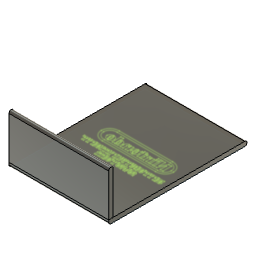
Nintendo Entertainment System Bookend (Autodesk Fusion 360 design; units mm, degrees)
Autodesk Fusion 360 part; units mm, degrees
sketch "Sketch1" plane through (0, 0, 0) normal (0, 0, 1) x (1, 0, 0)
  line L0 (0, 0) -> (67, 0)
  line L1 (67, 0) -> (67, 90)
  line L2 (67, 90) -> (0, 90)
  line L3 (0, 90) -> (0, 0)
  line L4 (0, 0) -> (67, 0)
  line L5 (67, 0) -> (67, -3)
  line L6 (67, -3) -> (0, -3)
  line L7 (0, -3) -> (0, 0)
  dimension "d1" = 67
  dimension "d2" = 90
  dimension "d3" = 67
  dimension "d4" = 3
  constraint horizontal L0
  constraint vertical L1
  constraint horizontal L2
  constraint vertical L3
  constraint coincident L0.start L3.end
  constraint horizontal L4
  constraint vertical L5
  constraint horizontal L6
  constraint vertical L7
  measures "d1" distance of L0.start L0.end
  measures "d2" distance of L0.start L2.end
  measures "d3" distance of L0.start L0.end
  measures "d4" distance of L0.start L6.end
extrude "Extrude1" add sketch "Sketch1" against normal blind 3 makes body 1
extrude "Extrude2" add sketch "Sketch1" along normal blind 30 separate body contours L0 L4 L5 L6 L7 makes body 2
fillet "Fillet1" radius 1.5 1 edges at (33.5, -3, -3) on bodies 1
fillet "Fillet2" radius 1.5 3 edges at (33.5, 90, -3) (33.5, -3, 30) (33.5, 0, 30) on bodies 1 2
fillet "Fillet3" radius 1.5 1 edges at (33.5, 90, 0) on bodies 1
sketch "Sketch2" plane through (0, 0, -3) normal (0, 0, -1) x (1, 0, 0)
  line L0 (0, -88.5) -> (67, -88.5)
  line L1 (67, -88.5) -> (67, 1.5)
  line L2 (67, 1.5) -> (0, 1.5)
  line L3 (0, 1.5) -> (0, -88.5)
  line L4 (53.2046, -41.1196) -> (56.3109, -41.1196)
  line L5 (56.3109, -41.1196) -> (56.3109, -38.078)
  line L6 (56.3109, -38.078) -> (55.3464, -38.078)
  line L7 (55.3464, -38.078) -> (55.3464, -40.1128)
  spline S0 degree 3 poles (55.3464, -40.1128) (55.3464, -40.2417) (55.2397, -40.3486) (55.111, -40.3486) knots 0 0 0 0 1 1 1 1
  line L8 (55.111, -40.3486) -> (53.4406, -40.3486)
  spline S1 degree 3 poles (53.4406, -40.3486) (53.3124, -40.3486) (53.2046, -40.2417) (53.2046, -40.1128) knots 0 0 0 0 1 1 1 1
  line L9 (53.2046, -40.1128) -> (53.2046, -38.078)
  line L10 (53.2046, -38.078) -> (52.2413, -38.078)
  line L11 (52.2413, -38.078) -> (52.2413, -40.1128)
  spline S2 degree 2 poles (52.2413, -40.1128) (52.1124, -41.1196) (53.2046, -41.1196) knots 0 0 0 1 1 1
  line L12 (26.3683, -41.1196) -> (29.4748, -41.1196)
  line L13 (29.4748, -41.1196) -> (29.4748, -38.078)
  line L14 (29.4748, -38.078) -> (28.4897, -38.078)
  line L15 (28.4897, -38.078) -> (28.4897, -40.1128)
  spline S3 degree 3 poles (28.4897, -40.1128) (28.4897, -40.2417) (28.3819, -40.3486) (28.2749, -40.3486) knots 0 0 0 0 1 1 1 1
  line L16 (28.2749, -40.3486) -> (26.6038, -40.3486)
  spline S4 degree 3 poles (26.6038, -40.3486) (26.4759, -40.3486) (26.3683, -40.2417) (26.3683, -40.1128) knots 0 0 0 0 1 1 1 1
  line L17 (26.3683, -40.1128) -> (26.3683, -38.078)
  line L18 (26.3683, -38.078) -> (25.4052, -38.078)
  line L19 (25.4052, -38.078) -> (25.4052, -40.1128)
  spline S5 degree 2 poles (25.4052, -40.1128) (25.2768, -41.1196) (26.3683, -41.1196) knots 0 0 0 1 1 1
  line L20 (11.74, -41.1196) -> (14.846, -41.1196)
  line L21 (14.846, -41.1196) -> (14.846, -38.078)
  line L22 (14.846, -38.078) -> (13.8814, -38.078)
  line L23 (13.8814, -38.078) -> (13.8814, -40.1128)
  spline S6 degree 3 poles (13.8814, -40.1128) (13.8814, -40.2417) (13.7753, -40.3486) (13.6459, -40.3486) knots 0 0 0 0 1 1 1 1
  line L24 (13.6459, -40.3486) -> (11.9756, -40.3486)
  spline S7 degree 3 poles (11.9756, -40.3486) (11.8477, -40.3486) (11.74, -40.2417) (11.74, -40.1128) knots 0 0 0 0 1 1 1 1
  line L25 (11.74, -40.1128) -> (11.74, -38.078)
  line L26 (11.74, -38.078) -> (10.7763, -38.078)
  line L27 (10.7763, -38.078) -> (10.7763, -40.1128)
  spline S8 degree 2 poles (10.7763, -40.1128) (10.6485, -41.1196) (11.74, -41.1196) knots 0 0 0 1 1 1
  line L28 (51.8126, -40.3486) -> (50.7419, -40.3486)
  spline S9 degree 3 poles (50.7419, -40.3486) (50.6348, -40.3486) (50.5059, -40.2417) (50.5059, -40.1128) knots 0 0 0 0 1 1 1 1
  line L29 (50.5059, -40.1128) -> (50.5059, -38.078)
  line L30 (50.5059, -38.078) -> (49.4786, -38.078)
  line L31 (49.4786, -38.078) -> (49.4786, -40.1128)
  spline S10 degree 3 poles (49.4786, -40.1128) (49.4786, -40.2417) (49.3709, -40.3486) (49.2427, -40.3486) knots 0 0 0 0 1 1 1 1
  line L32 (49.2427, -40.3486) -> (48.172, -40.3486)
  line L33 (48.172, -40.3486) -> (48.172, -41.1196)
  line L34 (48.172, -41.1196) -> (51.8126, -41.1196)
  line L35 (51.8126, -41.1196) -> (51.8126, -40.3486)
  line L36 (10.3698, -41.1196) -> (10.3698, -40.3486)
  line L37 (10.3698, -40.3486) -> (9.2984, -40.3486)
  spline S11 degree 3 poles (9.2984, -40.3486) (9.1706, -40.3486) (9.0628, -40.2417) (9.0628, -40.1128) knots 0 0 0 0 1 1 1 1
  line L38 (9.0628, -40.1128) -> (9.0628, -38.078)
  line L39 (9.0628, -38.078) -> (7.9914, -38.078)
  line L40 (7.9914, -38.078) -> (7.9914, -40.1128)
  spline S12 degree 3 poles (7.9914, -40.1128) (7.9914, -40.2417) (7.9067, -40.3486) (7.7782, -40.3486) knots 0 0 0 0 1 1 1 1
  line L41 (7.7782, -40.3486) -> (6.7068, -40.3486)
  line L42 (6.7068, -40.3486) -> (6.7068, -41.1196)
  line L43 (6.7068, -41.1196) -> (10.3698, -41.1196)
  line L44 (39.5829, -40.3486) -> (38.5121, -40.3486)
  spline S13 degree 3 poles (38.5121, -40.3486) (38.3839, -40.3486) (38.2763, -40.2417) (38.2763, -40.1128) knots 0 0 0 0 1 1 1 1
  line L45 (38.2763, -40.1128) -> (38.2763, -38.078)
  line L46 (38.2763, -38.078) -> (37.2063, -38.078)
  line L47 (37.2063, -38.078) -> (37.2063, -40.1128)
  spline S14 degree 3 poles (37.2063, -40.1128) (37.2063, -40.2417) (37.0985, -40.3486) (36.9696, -40.3486) knots 0 0 0 0 1 1 1 1
  line L48 (36.9696, -40.3486) -> (35.8996, -40.3486)
  line L49 (35.8996, -40.3486) -> (35.8996, -41.1196)
  line L50 (35.8996, -41.1196) -> (39.5829, -41.1196)
  line L51 (39.5829, -41.1196) -> (39.5829, -40.3486)
  line L52 (31.1446, -41.1196) -> (30.1168, -41.1196)
  line L53 (30.1168, -41.1196) -> (30.1168, -38.0781)
  line L54 (30.1168, -38.0781) -> (31.1446, -38.0781)
  line L55 (31.1446, -38.0781) -> (31.1446, -41.1196)
  line L56 (32.7941, -39.6198) -> (34.528, -39.6198)
  line L57 (34.528, -39.6198) -> (34.528, -40.1555)
  spline S15 degree 3 poles (34.528, -40.1555) (34.528, -40.2417) (34.3998, -40.3486) (34.3359, -40.3486) knots 0 0 0 0 1 1 1 1
  line L58 (34.3359, -40.3486) -> (33.0296, -40.3486)
  spline S16 degree 3 poles (33.0296, -40.3486) (32.8802, -40.3486) (32.7941, -40.2417) (32.7941, -40.1555) knots 0 0 0 0 1 1 1 1
  line L59 (32.7941, -40.1555) -> (32.7941, -39.6198)
  line L60 (32.8156, -41.1196) -> (34.5075, -41.1196)
  spline S17 degree 2 poles (34.5075, -41.1196) (35.5998, -41.1196) (35.5136, -40.1128) knots 0 0 0 1 1 1
  line L61 (35.5136, -40.1128) -> (35.5136, -38.078)
  line L62 (35.5136, -38.078) -> (34.528, -38.078)
  line L63 (34.528, -38.078) -> (34.528, -38.8485)
  line L64 (34.528, -38.8485) -> (32.7941, -38.8485)
  line L65 (32.7941, -38.8485) -> (32.7941, -38.078)
  line L66 (32.7941, -38.078) -> (31.8095, -38.078)
  line L67 (31.8095, -38.078) -> (31.8095, -40.1128)
  spline S18 degree 2 poles (31.8095, -40.1128) (31.681, -41.1196) (32.8156, -41.1196) knots 0 0 0 1 1 1
  spline S19 degree 3 poles (40.9539, -39.8553) (40.9539, -39.706) (41.0177, -39.6198) (41.1466, -39.6198) knots 0 0 0 0 1 1 1 1
  line L68 (41.1466, -39.6198) -> (42.5603, -39.6198)
  spline S20 degree 3 poles (42.5603, -39.6198) (42.6242, -39.6198) (42.7096, -39.706) (42.7096, -39.8553) knots 0 0 0 0 1 1 1 1
  line L69 (42.7096, -39.8553) -> (42.7096, -40.1555)
  spline S21 degree 3 poles (42.7096, -40.1555) (42.7096, -40.2844) (42.6242, -40.3913) (42.496, -40.3913) knots 0 0 0 0 1 1 1 1
  line L70 (42.496, -40.3913) -> (41.1466, -40.3913)
  spline S22 degree 3 poles (41.1466, -40.3913) (41.0177, -40.3913) (40.9539, -40.3278) (40.9539, -40.1555) knots 0 0 0 0 1 1 1 1
  line L71 (40.9539, -40.1555) -> (40.9539, -39.8553)
  line L72 (40.975, -41.1196) -> (43.7165, -41.1196)
  line L73 (43.7165, -41.1196) -> (43.7165, -38.078)
  line L74 (43.7165, -38.078) -> (42.7096, -38.078)
  line L75 (42.7096, -38.078) -> (42.7096, -38.6568)
  spline S23 degree 3 poles (42.7096, -38.6568) (42.7096, -38.7852) (42.6242, -38.8485) (42.496, -38.8485) knots 0 0 0 0 1 1 1 1
  line L76 (42.496, -38.8485) -> (41.1466, -38.8485)
  spline S24 degree 3 poles (41.1466, -38.8485) (41.0826, -38.8485) (40.9539, -38.7415) (40.9539, -38.6568) knots 0 0 0 0 1 1 1 1
  line L77 (40.9539, -38.6568) -> (40.9539, -38.078)
  line L78 (40.9539, -38.078) -> (39.9904, -38.078)
  line L79 (39.9904, -38.078) -> (39.9904, -38.5485)
  spline S25 degree 2 poles (39.9904, -38.5485) (39.9043, -38.9784) (40.3542, -39.2779) knots 0 0 0 1 1 1
  spline S26 degree 3 poles (40.3542, -39.2779) (40.0543, -39.4919) (39.947, -39.8123) (39.9255, -40.0061) knots 0 0 0 0 1 1 1 1
  spline S27 degree 2 poles (39.9255, -40.0061) (39.9043, -40.0916) (39.9043, -40.1555) knots 0 0 0 1 1 1
  spline S28 degree 2 poles (39.9043, -40.1555) (39.9043, -41.1196) (40.975, -41.1196) knots 0 0 0 1 1 1
  spline S29 degree 2 poles (60.3589, -39.0848) (60.4657, -38.078) (59.3518, -38.078) knots 0 0 0 1 1 1
  line L80 (59.3518, -38.078) -> (56.9529, -38.078)
  line L81 (56.9529, -38.078) -> (56.9529, -38.8485)
  line L82 (56.9529, -38.8485) -> (59.1808, -38.8485)
  spline S30 degree 3 poles (59.1808, -38.8485) (59.3306, -38.8485) (59.4595, -38.9784) (59.4595, -39.1057) knots 0 0 0 0 1 1 1 1
  spline S31 degree 3 poles (59.4595, -39.1057) (59.4595, -39.2556) (59.3518, -39.3418) (59.1808, -39.3418) knots 0 0 0 0 1 1 1 1
  line L83 (59.1808, -39.3418) -> (57.0811, -39.3418)
  line L84 (57.0811, -39.3418) -> (57.0811, -39.8769)
  line L85 (57.0811, -39.8769) -> (59.2236, -39.8769)
  spline S32 degree 3 poles (59.2236, -39.8769) (59.3518, -39.8769) (59.4595, -39.9839) (59.4595, -40.1128) knots 0 0 0 0 1 1 1 1
  spline S33 degree 3 poles (59.4595, -40.1128) (59.4595, -40.2417) (59.3518, -40.3486) (59.2236, -40.3486) knots 0 0 0 0 1 1 1 1
  line L86 (59.2236, -40.3486) -> (56.9529, -40.3486)
  line L87 (56.9529, -40.3486) -> (56.9529, -41.1196)
  line L88 (56.9529, -41.1196) -> (60.3589, -41.1196)
  line L89 (60.3589, -41.1196) -> (60.3589, -39.0848)
  spline S34 degree 2 poles (47.7217, -39.0848) (47.8722, -38.078) (46.7577, -38.078) knots 0 0 0 1 1 1
  line L90 (46.7577, -38.078) -> (44.3588, -38.078)
  line L91 (44.3588, -38.078) -> (44.3588, -38.8485)
  line L92 (44.3588, -38.8485) -> (46.5867, -38.8485)
  spline S35 degree 3 poles (46.5867, -38.8485) (46.7372, -38.8485) (46.8654, -38.9784) (46.8654, -39.1057) knots 0 0 0 0 1 1 1 1
  spline S36 degree 3 poles (46.8654, -39.1057) (46.8654, -39.2556) (46.7372, -39.3418) (46.5867, -39.3418) knots 0 0 0 0 1 1 1 1
  line L93 (46.5867, -39.3418) -> (44.4877, -39.3418)
  line L94 (44.4877, -39.3418) -> (44.4877, -39.8769)
  line L95 (44.4877, -39.8769) -> (46.5867, -39.8769)
  spline S37 degree 3 poles (46.5867, -39.8769) (46.7372, -39.8769) (46.8654, -39.9839) (46.8654, -40.1128) knots 0 0 0 0 1 1 1 1
  spline S38 degree 3 poles (46.8654, -40.1128) (46.8654, -40.2417) (46.7372, -40.3486) (46.5867, -40.3486) knots 0 0 0 0 1 1 1 1
  line L96 (46.5867, -40.3486) -> (44.3588, -40.3486)
  line L97 (44.3588, -40.3486) -> (44.3588, -41.1196)
  line L98 (44.3588, -41.1196) -> (47.7217, -41.1196)
  line L99 (47.7217, -41.1196) -> (47.7217, -39.0848)
  spline S39 degree 2 poles (18.8509, -39.0848) (18.9586, -38.078) (17.8656, -38.078) knots 0 0 0 1 1 1
  line L100 (17.8656, -38.078) -> (15.4456, -38.078)
  line L101 (15.4456, -38.078) -> (15.4456, -38.8485)
  line L102 (15.4456, -38.8485) -> (17.6948, -38.8485)
  spline S40 degree 3 poles (17.6948, -38.8485) (17.8232, -38.8485) (17.9517, -38.9784) (17.9517, -39.1057) knots 0 0 0 0 1 1 1 1
  spline S41 degree 3 poles (17.9517, -39.1057) (17.9517, -39.2556) (17.8656, -39.3418) (17.7156, -39.3418) knots 0 0 0 0 1 1 1 1
  line L103 (17.7156, -39.3418) -> (15.6172, -39.3418)
  line L104 (15.6172, -39.3418) -> (15.6172, -39.8769)
  line L105 (15.6172, -39.8769) -> (17.7156, -39.8769)
  spline S42 degree 3 poles (17.7156, -39.8769) (17.8656, -39.8769) (17.9517, -39.9839) (17.9517, -40.1128) knots 0 0 0 0 1 1 1 1
  spline S43 degree 3 poles (17.9517, -40.1128) (17.9517, -40.2417) (17.8656, -40.3486) (17.7156, -40.3486) knots 0 0 0 0 1 1 1 1
  line L106 (17.7156, -40.3486) -> (15.4456, -40.3486)
  line L107 (15.4456, -40.3486) -> (15.4456, -41.1196)
  line L108 (15.4456, -41.1196) -> (18.8509, -41.1196)
  line L109 (18.8509, -41.1196) -> (18.8509, -39.0848)
  line L110 (20.45, -41.1156) -> (24.7558, -41.1156)
  line L111 (24.7558, -41.1156) -> (24.7558, -38.0745)
  line L112 (24.7558, -38.0745) -> (23.856, -38.0745)
  line L113 (23.856, -38.0745) -> (23.856, -40.1088)
  spline S44 degree 3 poles (23.856, -40.1088) (23.856, -40.2369) (23.749, -40.3443) (23.6204, -40.3443) knots 0 0 0 0 1 1 1 1
  line L114 (23.6204, -40.3443) -> (22.8928, -40.3443)
  spline S45 degree 3 poles (22.8928, -40.3443) (22.7638, -40.3443) (22.6561, -40.2369) (22.6561, -40.1088) knots 0 0 0 0 1 1 1 1
  line L115 (22.6561, -40.1088) -> (22.6561, -38.0745)
  line L116 (22.6561, -38.0745) -> (21.6499, -38.0745)
  line L117 (21.6499, -38.0745) -> (21.6499, -40.1088)
  spline S46 degree 3 poles (21.6499, -40.1088) (21.6499, -40.2369) (21.5638, -40.3443) (21.4143, -40.3443) knots 0 0 0 0 1 1 1 1
  line L118 (21.4143, -40.3443) -> (20.643, -40.3443)
  spline S47 degree 3 poles (20.643, -40.3443) (20.5577, -40.3443) (20.45, -40.2369) (20.45, -40.1088) knots 0 0 0 0 1 1 1 1
  line L119 (20.45, -40.1088) -> (20.4082, -38.0745)
  line L120 (20.4082, -38.0745) -> (19.4445, -38.0745)
  line L121 (19.4445, -38.0745) -> (19.4445, -40.1088)
  spline S48 degree 2 poles (19.4445, -40.1088) (19.316, -41.1156) (20.45, -41.1156) knots 0 0 0 1 1 1
  line L122 (34.143, -36.1081) -> (33.0511, -36.1081)
  spline S49 degree 3 poles (33.0511, -36.1081) (32.9664, -36.1081) (32.8587, -36.0004) (32.8587, -35.8726) knots 0 0 0 0 1 1 1 1
  line L123 (32.8587, -35.8726) -> (32.8587, -33.8382)
  line L124 (32.8587, -33.8382) -> (31.7872, -33.8382)
  line L125 (31.7872, -33.8382) -> (31.7448, -35.8726)
  spline S50 degree 3 poles (31.7448, -35.8726) (31.7448, -36.0004) (31.681, -36.1081) (31.5517, -36.1081) knots 0 0 0 0 1 1 1 1
  line L126 (31.5517, -36.1081) -> (30.4803, -36.1081)
  line L127 (30.4803, -36.1081) -> (30.4803, -36.8787)
  line L128 (30.4803, -36.8787) -> (34.143, -36.8787)
  line L129 (34.143, -36.8787) -> (34.143, -36.1081)
  line L130 (21.7636, -36.8787) -> (26.0681, -36.8787)
  line L131 (26.0681, -36.8787) -> (26.0681, -33.8382)
  line L132 (26.0681, -33.8382) -> (25.169, -33.8382)
  line L133 (25.169, -33.8382) -> (25.169, -35.8726)
  spline S51 degree 3 poles (25.169, -35.8726) (25.169, -36.0004) (25.062, -36.1081) (24.9334, -36.1081) knots 0 0 0 0 1 1 1 1
  line L134 (24.9334, -36.1081) -> (24.2053, -36.1081)
  spline S52 degree 3 poles (24.2053, -36.1081) (24.0774, -36.1081) (23.9704, -36.0004) (23.9704, -35.8726) knots 0 0 0 0 1 1 1 1
  line L135 (23.9704, -35.8726) -> (23.9704, -33.8382)
  line L136 (23.9704, -33.8382) -> (22.9637, -33.8382)
  line L137 (22.9637, -33.8382) -> (22.9637, -35.8726)
  spline S53 degree 3 poles (22.9637, -35.8726) (22.9637, -36.0004) (22.8781, -36.1081) (22.7274, -36.1081) knots 0 0 0 0 1 1 1 1
  line L138 (22.7274, -36.1081) -> (21.9568, -36.1081)
  spline S54 degree 3 poles (21.9568, -36.1081) (21.8707, -36.1081) (21.7636, -36.0004) (21.7636, -35.8726) knots 0 0 0 0 1 1 1 1
  line L139 (21.7636, -35.8726) -> (21.7206, -33.8382)
  line L140 (21.7206, -33.8382) -> (20.7568, -33.8382)
  line L141 (20.7568, -33.8382) -> (20.7568, -35.8726)
  spline S55 degree 2 poles (20.7568, -35.8726) (20.629, -36.8787) (21.7636, -36.8787) knots 0 0 0 1 1 1
  line L142 (38.5549, -36.8787) -> (39.4762, -36.8787)
  line L143 (39.4762, -36.8787) -> (39.4762, -35.7434)
  spline S56 degree 3 poles (39.4762, -35.7434) (39.4762, -35.6161) (39.6044, -35.5085) (39.7111, -35.5085) knots 0 0 0 0 1 1 1 1
  line L144 (39.7111, -35.5085) -> (41.0826, -35.5085)
  spline S57 degree 3 poles (41.0826, -35.5085) (41.2108, -35.5085) (41.3182, -35.6161) (41.3182, -35.7434) knots 0 0 0 0 1 1 1 1
  line L145 (41.3182, -35.7434) -> (41.3182, -36.8787)
  line L146 (41.3182, -36.8787) -> (42.2816, -36.8787)
  line L147 (42.2816, -36.8787) -> (42.2816, -35.7649)
  spline S58 degree 2 poles (42.2816, -35.7649) (42.3886, -34.7379) (41.2748, -34.7379) knots 0 0 0 1 1 1
  line L148 (41.2748, -34.7379) -> (40.9539, -34.7379)
  line L149 (40.9539, -34.7379) -> (40.9539, -33.8382)
  line L150 (40.9539, -33.8382) -> (39.8827, -33.8382)
  line L151 (39.8827, -33.8382) -> (39.8827, -34.7379)
  line L152 (39.8827, -34.7379) -> (39.5189, -34.7379)
  spline S59 degree 2 poles (39.5189, -34.7379) (38.4051, -34.7379) (38.5549, -35.7434) knots 0 0 0 1 1 1
  line L153 (38.5549, -35.7434) -> (38.5549, -36.8787)
  spline S60 degree 2 poles (30.0739, -34.8443) (30.2238, -33.8382) (29.1101, -33.8382) knots 0 0 0 1 1 1
  line L154 (29.1101, -33.8382) -> (26.7115, -33.8382)
  line L155 (26.7115, -33.8382) -> (26.7115, -34.6093)
  line L156 (26.7115, -34.6093) -> (28.9385, -34.6093)
  spline S61 degree 3 poles (28.9385, -34.6093) (29.0886, -34.6093) (29.2177, -34.7164) (29.2177, -34.8665) knots 0 0 0 0 1 1 1 1
  spline S62 degree 3 poles (29.2177, -34.8665) (29.2177, -35.0158) (29.0886, -35.0797) (28.9385, -35.0797) knots 0 0 0 0 1 1 1 1
  line L157 (28.9385, -35.0797) -> (26.8401, -35.0797)
  line L158 (26.8401, -35.0797) -> (26.8401, -35.6161)
  line L159 (26.8401, -35.6161) -> (28.9385, -35.6161)
  spline S63 degree 3 poles (28.9385, -35.6161) (29.0886, -35.6161) (29.2177, -35.7434) (29.2177, -35.8726) knots 0 0 0 0 1 1 1 1
  spline S64 degree 3 poles (29.2177, -35.8726) (29.2177, -36.0004) (29.0886, -36.1081) (28.9385, -36.1081) knots 0 0 0 0 1 1 1 1
  line L160 (28.9385, -36.1081) -> (26.7115, -36.1081)
  line L161 (26.7115, -36.1081) -> (26.7115, -36.8787)
  line L162 (26.7115, -36.8787) -> (30.0739, -36.8787)
  line L163 (30.0739, -36.8787) -> (30.0739, -34.8443)
  line L164 (35.4709, -35.6377) -> (36.9064, -35.6377)
  spline S65 degree 3 poles (36.9064, -35.6377) (37.0773, -35.6377) (37.184, -35.701) (37.184, -35.8504) knots 0 0 0 0 1 1 1 1
  spline S66 degree 3 poles (37.184, -35.8504) (37.184, -35.9802) (37.0773, -36.1081) (36.9491, -36.1081) knots 0 0 0 0 1 1 1 1
  line L165 (36.9491, -36.1081) -> (34.5075, -36.1081)
  line L166 (34.5075, -36.1081) -> (34.5075, -36.8787)
  line L167 (34.5075, -36.8787) -> (37.184, -36.8787)
  spline S67 degree 3 poles (37.184, -36.8787) (37.677, -36.8787) (38.1047, -36.4722) (38.1047, -36.0004) knots 0 0 0 0 1 1 1 1
  spline S68 degree 3 poles (38.1047, -36.0004) (38.1047, -35.3368) (37.677, -35.0797) (37.0985, -35.0797) knots 0 0 0 0 1 1 1 1
  line L168 (37.0985, -35.0797) -> (35.6637, -35.0797)
  spline S69 degree 3 poles (35.6637, -35.0797) (35.5136, -35.0797) (35.3636, -35.0158) (35.3636, -34.8665) knots 0 0 0 0 1 1 1 1
  spline S70 degree 3 poles (35.3636, -34.8665) (35.3636, -34.7379) (35.4709, -34.6093) (35.5998, -34.6093) knots 0 0 0 0 1 1 1 1
  line L169 (35.5998, -34.6093) -> (38.1047, -34.6093)
  line L170 (38.1047, -34.6093) -> (38.1047, -33.8382)
  line L171 (38.1047, -33.8382) -> (35.3636, -33.8382)
  spline S71 degree 3 poles (35.3636, -33.8382) (34.914, -33.8382) (34.4426, -34.2022) (34.4426, -34.7164) knots 0 0 0 0 1 1 1 1
  spline S72 degree 3 poles (34.4426, -34.7164) (34.4426, -35.3368) (34.9356, -35.6377) (35.4709, -35.6377) knots 0 0 0 0 1 1 1 1
  line L172 (43.631, -35.6377) -> (45.023, -35.6377)
  spline S73 degree 3 poles (45.023, -35.6377) (45.1947, -35.6377) (45.3229, -35.701) (45.3229, -35.8504) knots 0 0 0 0 1 1 1 1
  spline S74 degree 3 poles (45.3229, -35.8504) (45.3229, -35.9802) (45.1947, -36.1081) (45.0658, -36.1081) knots 0 0 0 0 1 1 1 1
  line L173 (45.0658, -36.1081) -> (42.6242, -36.1081)
  line L174 (42.6242, -36.1081) -> (42.6242, -36.8787)
  line L175 (42.6242, -36.8787) -> (45.3017, -36.8787)
  spline S75 degree 3 poles (45.3017, -36.8787) (45.8371, -36.8787) (46.2657, -36.4722) (46.2657, -36.0004) knots 0 0 0 0 1 1 1 1
  spline S76 degree 3 poles (46.2657, -36.0004) (46.2657, -35.3368) (45.7943, -35.0797) (45.2162, -35.0797) knots 0 0 0 0 1 1 1 1
  line L176 (45.2162, -35.0797) -> (43.8241, -35.0797)
  spline S77 degree 3 poles (43.8241, -35.0797) (43.6525, -35.0797) (43.5243, -35.0158) (43.5243, -34.8665) knots 0 0 0 0 1 1 1 1
  spline S78 degree 3 poles (43.5243, -34.8665) (43.5243, -34.7379) (43.6525, -34.6093) (43.7813, -34.6093) knots 0 0 0 0 1 1 1 1
  line L177 (43.7813, -34.6093) -> (46.2657, -34.6093)
  line L178 (46.2657, -34.6093) -> (46.2657, -33.8382)
  line L179 (46.2657, -33.8382) -> (43.5243, -33.8382)
  spline S79 degree 3 poles (43.5243, -33.8382) (43.0316, -33.8382) (42.5814, -34.2022) (42.5814, -34.7164) knots 0 0 0 0 1 1 1 1
  spline S80 degree 3 poles (42.5814, -34.7164) (42.5814, -35.3368) (43.0529, -35.6377) (43.631, -35.6377) knots 0 0 0 0 1 1 1 1
  spline S81 degree 3 poles (51.5861, -43.9141) (55.3819, -43.9152) (57.9183, -46.4889) (57.9183, -49.6094) knots 0 0 0 0 1 1 1 1
  spline S82 degree 3 poles (57.9183, -49.6094) (57.9183, -52.7298) (55.3761, -55.3329) (51.5919, -55.3249) knots 0 0 0 0 1 1 1 1
  line L180 (51.5919, -55.3249) -> (15.8311, -55.3249)
  spline S83 degree 3 poles (15.8311, -55.3249) (12.0469, -55.3329) (9.5047, -52.7298) (9.5047, -49.6094) knots 0 0 0 0 1 1 1 1
  spline S84 degree 3 poles (9.5047, -49.6094) (9.5047, -46.4889) (12.0411, -43.9153) (15.8369, -43.9141) knots 0 0 0 0 1 1 1 1
  line L181 (15.8369, -43.9141) -> (51.5861, -43.9141)
  spline S85 degree 3 poles (51.5745, -53.9213) (54.5795, -53.9158) (56.4241, -51.9941) (56.4241, -49.6168) knots 0 0 0 0 1 1 1 1
  spline S86 degree 3 poles (56.4241, -49.6168) (56.4241, -47.24) (54.5911, -45.3024) (51.5745, -45.3129) knots 0 0 0 0 1 1 1 1
  line L182 (51.5745, -45.3129) -> (15.8485, -45.3129)
  spline S87 degree 3 poles (15.8485, -45.3129) (12.8319, -45.303) (10.9982, -47.24) (10.9982, -49.6168) knots 0 0 0 0 1 1 1 1
  spline S88 degree 3 poles (10.9982, -49.6168) (10.9982, -51.9935) (12.8428, -53.9151) (15.8478, -53.9207) knots 0 0 0 0 1 1 1 1
  line L183 (15.8478, -53.9207) -> (51.5745, -53.9213)
  line L184 (49.5717, -52.4118) -> (47.8083, -52.4118)
  line L185 (47.8083, -52.4118) -> (47.8083, -46.7083)
  line L186 (47.8083, -46.7083) -> (49.5691, -46.7083)
  line L187 (49.5691, -46.7083) -> (52.0404, -50.6856)
  line L188 (52.0404, -50.6856) -> (52.0404, -46.7083)
  line L189 (52.0404, -46.7083) -> (53.8064, -46.7083)
  line L190 (53.8064, -46.7083) -> (53.8057, -52.4118)
  line L191 (53.8057, -52.4118) -> (52.0287, -52.4118)
  line L192 (52.0287, -52.4118) -> (49.5704, -48.4344)
  line L193 (49.5704, -48.4344) -> (49.5717, -52.4118)
  line L194 (39.1541, -50.4936) -> (39.1541, -51.0566)
  line L195 (39.1541, -51.0566) -> (38.2208, -51.0573)
  line L196 (38.2208, -51.0573) -> (38.2221, -51.8253)
  line L197 (38.2221, -51.8253) -> (36.5058, -51.8253)
  line L198 (36.5058, -51.8253) -> (36.5058, -51.0579)
  line L199 (36.5058, -51.0579) -> (35.5771, -51.0579)
  line L200 (35.5771, -51.0579) -> (35.5771, -50.4936)
  line L201 (35.5771, -50.4936) -> (36.5058, -50.4936)
  line L202 (36.5058, -50.4936) -> (36.5045, -46.7083)
  line L203 (36.5045, -46.7083) -> (38.2221, -46.7083)
  line L204 (38.2221, -46.7083) -> (38.2215, -50.4936)
  line L205 (38.2215, -50.4936) -> (39.1541, -50.4936)
  line L206 (45.1117, -50.5008) -> (45.1117, -46.7083)
  line L207 (45.1117, -46.7083) -> (46.8267, -46.7083)
  line L208 (46.8267, -46.7083) -> (46.8267, -50.5015)
  line L209 (46.8267, -50.5015) -> (45.1117, -50.5008)
  line L210 (45.1117, -52.4131) -> (45.1117, -51.2473)
  line L211 (45.1117, -51.2473) -> (46.8306, -51.2473)
  line L212 (46.8306, -51.2473) -> (46.8306, -52.4131)
  line L213 (46.8306, -52.4131) -> (45.1117, -52.4131)
  spline S89 degree 2 poles (16.0814, -48.6349) (16.0822, -48.0615) (16.0822, -47.8316) knots 0 0 0 1 1 1
  spline S90 degree 3 poles (16.0822, -47.8316) (16.0822, -47.2268) (16.4394, -46.9773) (16.783, -46.9773) knots 0 0 0 0 1 1 1 1
  spline S91 degree 3 poles (16.783, -46.9773) (17.1272, -46.9773) (17.4857, -47.2268) (17.4857, -47.8316) knots 0 0 0 0 1 1 1 1
  spline S92 degree 2 poles (17.4857, -47.8316) (17.4857, -48.0615) (17.485, -48.6493) knots 0 0 0 1 1 1
  spline S93 degree 2 poles (17.485, -48.6493) (17.4837, -49.2103) (17.4837, -49.4402) knots 0 0 0 1 1 1
  spline S94 degree 3 poles (17.4837, -49.4402) (17.4837, -50.0423) (17.1245, -50.2899) (16.7829, -50.2899) knots 0 0 0 0 1 1 1 1
  spline S95 degree 3 poles (16.7829, -50.2899) (16.4407, -50.2899) (16.0822, -50.0423) (16.0822, -49.4402) knots 0 0 0 0 1 1 1 1
  spline S96 degree 3 poles (16.0822, -49.4402) (16.0822, -49.2103) (16.0829, -48.7851) (16.0809, -48.633) knots 0 0 0 0 1 1 1 1
  line L214 (16.0809, -48.633) -> (16.0814, -48.6349)
  spline S97 degree 3 poles (16.7705, -50.7601) (18.155, -50.7601) (19.2771, -49.8066) (19.2771, -48.6303) knots 0 0 0 0 1 1 1 1
  spline S98 degree 3 poles (19.2771, -48.6303) (19.2771, -47.4541) (18.1544, -46.5006) (16.7705, -46.5006) knots 0 0 0 0 1 1 1 1
  spline S99 degree 3 poles (16.7705, -46.5006) (15.3859, -46.5006) (14.2639, -47.4541) (14.2639, -48.6303) knots 0 0 0 0 1 1 1 1
  spline S100 degree 3 poles (14.2639, -48.6303) (14.2639, -49.8066) (15.3859, -50.7601) (16.7705, -50.7601) knots 0 0 0 0 1 1 1 1
  line L215 (21.5283, -52.4118) -> (19.8355, -52.4118)
  line L216 (19.8355, -52.4118) -> (19.8355, -46.7083)
  line L217 (19.8355, -46.7083) -> (21.5309, -46.7083)
  spline S101 degree 2 poles (21.5309, -46.7083) (21.5317, -46.8924) (21.5317, -46.9277) knots 0 0 0 1 1 1
  spline S102 degree 3 poles (21.5317, -46.9277) (22.188, -46.5156) (22.9286, -46.5163) (23.5053, -46.7853) knots 0 0 0 0 1 1 1 1
  spline S103 degree 3 poles (23.5053, -46.7853) (23.6601, -46.8572) (24.6783, -47.3457) (24.6783, -48.6656) knots 0 0 0 0 1 1 1 1
  spline S104 degree 3 poles (24.6783, -48.6656) (24.6783, -49.6668) (23.7339, -50.7601) (22.4976, -50.6517) knots 0 0 0 0 1 1 1 1
  spline S105 degree 3 poles (22.4976, -50.6517) (22.0907, -50.6158) (21.8014, -50.4675) (21.5271, -50.3134) knots 0 0 0 0 1 1 1 1
  spline S106 degree 2 poles (21.5271, -50.3134) (21.5283, -51.1911) (21.5283, -52.4118) knots 0 0 0 1 1 1
  spline S107 degree 2 poles (21.5159, -48.6238) (21.5159, -49.0993) (21.5159, -49.3017) knots 0 0 0 1 1 1
  spline S108 degree 3 poles (21.5159, -49.3017) (21.5159, -49.8882) (21.9208, -50.0378) (22.1873, -50.0378) knots 0 0 0 0 1 1 1 1
  spline S109 degree 3 poles (22.1873, -50.0378) (22.4603, -50.0378) (22.86, -49.8882) (22.86, -49.3017) knots 0 0 0 0 1 1 1 1
  spline S110 degree 2 poles (22.86, -49.3017) (22.86, -49.1071) (22.8592, -48.6258) knots 0 0 0 1 1 1
  spline S111 degree 2 poles (22.8592, -48.6258) (22.86, -48.1529) (22.86, -47.9511) knots 0 0 0 1 1 1
  spline S112 degree 3 poles (22.86, -47.9511) (22.86, -47.3653) (22.4603, -47.2118) (22.1879, -47.2118) knots 0 0 0 0 1 1 1 1
  spline S113 degree 3 poles (22.1879, -47.2118) (21.9208, -47.2118) (21.5152, -47.3653) (21.5152, -47.9511) knots 0 0 0 0 1 1 1 1
  spline S114 degree 2 poles (21.5152, -47.9511) (21.5152, -48.1947) (21.5159, -48.6238) knots 0 0 0 1 1 1
  spline S115 degree 3 poles (41.0964, -50.6765) (40.4551, -50.6948) (39.1541, -50.2748) (39.1633, -48.7734) knots 0 0 0 0 1 1 1 1
  spline S116 degree 2 poles (39.1633, -48.7734) (39.1646, -48.5069) (39.1639, -46.7096) knots 0 0 0 1 1 1
  line L218 (39.1639, -46.7096) -> (40.8678, -46.7096)
  spline S117 degree 2 poles (40.8678, -46.7096) (40.8678, -48.9634) (40.8678, -49.2005) knots 0 0 0 1 1 1
  spline S118 degree 3 poles (40.8678, -49.2005) (40.8678, -49.531) (41.1839, -49.8987) (41.6516, -49.8987) knots 0 0 0 0 1 1 1 1
  spline S119 degree 3 poles (41.6516, -49.8987) (42.1185, -49.8987) (42.466, -49.531) (42.466, -49.2005) knots 0 0 0 0 1 1 1 1
  spline S120 degree 2 poles (42.466, -49.2005) (42.466, -49.0385) (42.464, -46.7096) knots 0 0 0 1 1 1
  line L219 (42.464, -46.7096) -> (44.1667, -46.7096)
  line L220 (44.1667, -46.7096) -> (44.1673, -50.5021)
  line L221 (44.1673, -50.5021) -> (42.4634, -50.5034)
  spline S121 degree 2 poles (42.4634, -50.5034) (42.4653, -50.1984) (42.4634, -50.1044) knots 0 0 0 1 1 1
  spline S122 degree 3 poles (42.4634, -50.1044) (42.1355, -50.4172) (41.6633, -50.6602) (41.0964, -50.6765) knots 0 0 0 0 1 1 1 1
  spline S123 degree 3 poles (27.158, -50.6765) (26.5167, -50.6948) (25.2157, -50.2748) (25.2248, -48.7734) knots 0 0 0 0 1 1 1 1
  spline S124 degree 2 poles (25.2248, -48.7734) (25.2261, -48.5069) (25.2256, -46.7096) knots 0 0 0 1 1 1
  line L222 (25.2256, -46.7096) -> (26.9295, -46.7096)
  spline S125 degree 2 poles (26.9295, -46.7096) (26.9295, -48.9634) (26.9295, -49.2005) knots 0 0 0 1 1 1
  spline S126 degree 3 poles (26.9295, -49.2005) (26.9295, -49.531) (27.2456, -49.8987) (27.7132, -49.8987) knots 0 0 0 0 1 1 1 1
  spline S127 degree 3 poles (27.7132, -49.8987) (28.1802, -49.8987) (28.5276, -49.531) (28.5276, -49.2005) knots 0 0 0 0 1 1 1 1
  spline S128 degree 2 poles (28.5276, -49.2005) (28.5276, -49.0385) (28.5257, -46.7096) knots 0 0 0 1 1 1
  line L223 (28.5257, -46.7096) -> (30.2283, -46.7096)
  line L224 (30.2283, -46.7096) -> (30.227, -50.5021)
  line L225 (30.227, -50.5021) -> (28.5251, -50.5034)
  spline S129 degree 2 poles (28.5251, -50.5034) (28.5271, -50.1984) (28.5251, -50.1044) knots 0 0 0 1 1 1
  spline S130 degree 3 poles (28.5251, -50.1044) (28.1972, -50.4172) (27.7244, -50.6602) (27.158, -50.6765) knots 0 0 0 0 1 1 1 1
  spline S131 degree 3 poles (33.9796, -49.1789) (33.9822, -49.5114) (33.975, -49.7334) (33.866, -49.9228) knots 0 0 0 0 1 1 1 1
  spline S132 degree 3 poles (33.866, -49.9228) (33.7321, -50.1566) (33.4859, -50.2677) (33.2625, -50.269) knots 0 0 0 0 1 1 1 1
  spline S133 degree 3 poles (33.2625, -50.269) (33.0399, -50.2677) (32.7937, -50.1566) (32.6598, -49.9228) knots 0 0 0 0 1 1 1 1
  spline S134 degree 3 poles (32.6598, -49.9228) (32.5507, -49.7328) (32.5462, -49.5107) (32.5488, -49.1783) knots 0 0 0 0 1 1 1 1
  line L226 (32.5488, -49.1783) -> (33.9796, -49.1789)
  spline S135 degree 2 poles (32.5546, -48.0354) (32.5533, -48.0184) (32.5533, -47.8055) knots 0 0 0 1 1 1
  spline S136 degree 3 poles (32.5533, -47.8055) (32.5533, -47.1119) (33.0098, -46.9578) (33.2632, -46.9578) knots 0 0 0 0 1 1 1 1
  spline S137 degree 3 poles (33.2632, -46.9578) (33.5166, -46.9578) (33.981, -47.1119) (33.981, -47.8055) knots 0 0 0 0 1 1 1 1
  spline S138 degree 2 poles (33.981, -47.8055) (33.981, -48.0132) (33.9797, -48.5885) knots 0 0 0 1 1 1
  spline S139 degree 2 poles (33.9797, -48.5885) (30.7489, -48.5872) (30.7489, -48.5892) knots 0 0 0 1 1 1
  spline S140 degree 3 poles (30.7489, -48.5892) (30.7489, -49.7654) (31.8846, -50.7398) (33.2796, -50.7398) knots 0 0 0 0 1 1 1 1
  spline S141 degree 3 poles (33.2796, -50.7398) (34.6746, -50.7398) (35.8051, -49.7863) (35.8051, -48.6101) knots 0 0 0 0 1 1 1 1
  spline S142 degree 3 poles (35.8051, -48.6101) (35.8051, -47.4339) (34.6746, -46.481) (33.2796, -46.481) knots 0 0 0 0 1 1 1 1
  spline S143 degree 3 poles (33.2796, -46.481) (32.1223, -46.481) (31.1446, -47.1413) (30.8462, -48.0367) knots 0 0 0 0 1 1 1 1
  line L227 (30.8462, -48.0367) -> (32.5546, -48.0354)
extrude "Extrude3" cut sketch "Sketch2" against normal blind 1 contours S81 S82 L180 S83 S84 L181 | L184 L185 L186 L187 L188 L189 L190 L191 L192 L193 | L194 L195 L196 L197 L198 L199 L200 L201 L202 L203 L204 L205 | L206 L207 L208 L209 | L210 L211 L212 L213 | S97 S98 S99 S100 | L215 L216 L217 S101 S102 S103 S104 S105 S106 | S115 S116 L218 S117 S118 S119 S120 L219 L220 L221 S121 S122 | S123 S124 L222 S125 S126 S127 S128 L223 L224 L225 S129 S130 | S135 S136 S137 S138 S139 S140 S141 S142 S143 L227 bodies 1
extrude "Extrude4" cut sketch "Sketch2" against normal blind 1 contours L4 L5 L6 L7 S0 L8 S1 L9 L10 L11 S2 | L12 L13 L14 L15 S3 L16 S4 L17 L18 L19 S5 | L20 L21 L22 L23 S6 L24 S7 L25 L26 L27 S8 | L28 S9 L29 L30 L31 S10 L32 L33 L34 L35 | L36 L37 S11 L38 L39 L40 S12 L41 L42 L43 | L44 S13 L45 L46 L47 S14 L48 L49 L50 L51 | L52 L53 L54 L55 | L60 S17 L61 L62 L63 L64 L65 L66 L67 S18 | L72 L73 L74 L75 S23 L76 S24 L77 L78 L79 S25 S26 S27 S28 | S29 L80 L81 L82 S30 S31 L83 L84 L85 S32 S33 L86 L87 L88 L89 | S34 L90 L91 L92 S35 S36 L93 L94 L95 S37 S38 L96 L97 L98 L99 | S39 L100 L101 L102 S40 S41 L103 L104 L105 S42 S43 L106 L107 L108 L109 | L110 L111 L112 L113 S44 L114 S45 L115 L116 L117 S46 L118 S47 L119 L120 L121 S48 | L122 S49 L123 L124 L125 S50 L126 L127 L128 L129 | L130 L131 L132 L133 S51 L134 S52 L135 L136 L137 S53 L138 S54 L139 L140 L141 S55 | L142 L143 S56 L144 S57 L145 L146 L147 S58 L148 L149 L150 L151 L152 S59 L153 | S60 L154 L155 L156 S61 S62 L157 L158 L159 S63 S64 L160 L161 L162 L163 | L164 S65 S66 L165 L166 L167 S67 S68 L168 S69 S70 L169 L170 L171 S71 S72 | L172 S73 S74 L173 L174 L175 S75 S76 L176 S77 S78 L177 L178 L179 S79 S80 bodies 1
